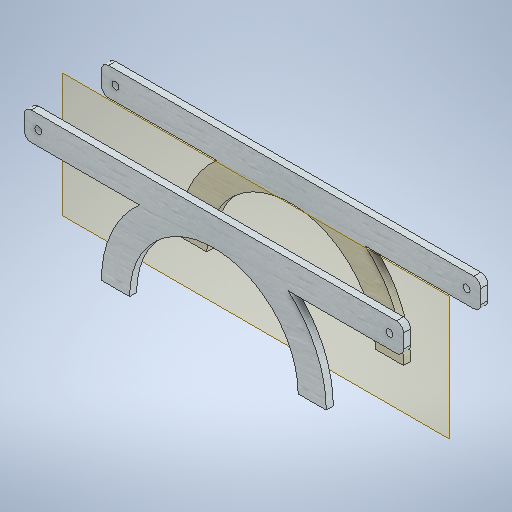
# Autodesk Inventor part: Conveyor_001_001
Saved by Autodesk Inventor 2026 (Build 300175000, 175)
## iProperties
Created: 2025-05-22
Part Number: Conveyor_001_001
Material: ABS Plastic
Document SubType Name: Modeling
Designer: carlo
Density: 1.06 g/cm^3
Appearance: Wood - Painted White
Author: carlo
Autodesk Inventor part; units mm, degrees
ref_plane "YZ Plane" through (0, 0, 0) normal (1, 0, 0) x (0, 1, 0)
ref_plane "XZ Plane" through (0, 0, 0) normal (0, 1, 0) x (-1, 0, 0)
ref_plane "XY Plane" through (0, 0, 0) normal (0, 0, 1) x (1, 0, 0)
sketch "Sketch1" plane through (0, 0, 0) normal (0, 0, 1) x (1, 0, 0)
  line L0 (-135, 80) -> (135, 80)
  line L1 (-135, 80) -> (-135, 60)
  line L2 (135, 80) -> (135, 60)
  line L3 (-135, 60) -> (135, 60)
  arc A0 (60, 0) -> (-60, 0) centre (0, 0) ccw
  arc A1 (80, 0) -> (-80, 0) centre (0, 0) ccw
  line L4 (80, 0) -> (60, 0)
  line L5 (60, 0) -> (80, 0)
  line L6 (-60, 0) -> (-80, 0)
  circle A2 centre (125, 70) radius 2.5
  circle A3 centre (-125, 70) radius 2.5
  point P0 (0, 80)
  point P1 (52.915, 60)
  point P2 (-52.915, 60)
  point P3 (-135, 70)
  point P4 (-125, 80)
  point P5 (-125, 60)
  point P6 (125, 60)
  point P7 (125, 80)
  point P8 (135, 70)
  point P9 (-135, 70)
  point P10 (0, 80)
  point P11 (0, 60)
  dimension "d0" = 270
  dimension "d1" = 80
  dimension "d2" = 20
  dimension "d10" = 5
  dimension "d11" = 10
  dimension "d12" = 10
  dimension "d13" = 5
  dimension "d14" = 10
  dimension "d15" = 10
  constraints: 14 end point, 5 horizontal, 4 centre point, 4 point on circle, 2 coincident, 2 horizontal alignment, 2 midpoint, 2 tangent, 2 vertical, 1 parallel, 1 vertical alignment
  measures "d0" distance of L0.start L0.end
  measures "d1" distance from line of point (0, 0) L0
  measures "d2" distance of L0.start L1.end
  measures "d10" diameter of A2
  measures "d11" distance from line of L0 A2.centre
  measures "d12" distance from line of L2 A2.centre
  measures "d13" diameter of A3
  measures "d14" distance from line of L0 A3.centre
  measures "d15" distance of point (-135, 70) A3.centre
extrude "Extrusion2" add sketch "Sketch1" along normal mid plane 5
ref_plane "Work Plane3" through (0, 0, 27.5) normal (0, 0, 1) x (1, 0, 0)
mirror "Mirror2" about plane through (0, 0, 27.5) normal (0, 0, 1) of "Extrusion2"
fillet "Fillet1" radius 5 8 edges at (135, 80, 0) (135, 60, 0) (135, 80, 55) (135, 60, 55) (-135, 80, 0) (-135, 60, 0) (-135, 80, 55) (-135, 60, 55)
body "Solid2"
